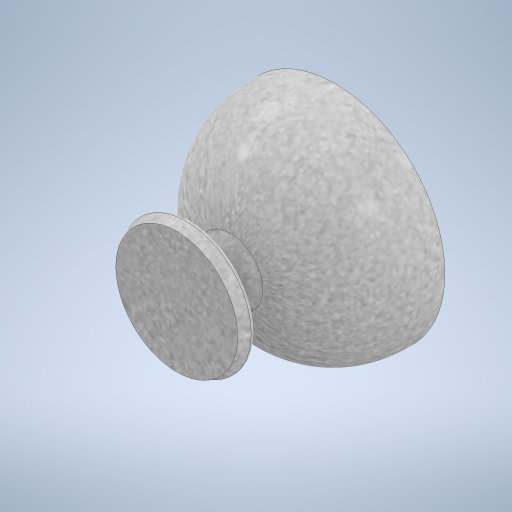
# Autodesk Inventor part: icecup
Saved by Autodesk Inventor 2024 (Build 280153000, 153)
## iProperties
Created: 2024-03-22
Part Number: icecup
Material: Glasfaserbeton
Document SubType Name: Modeling
Designer: ffogue
Density: 1.7 g/cm^3
Appearance: Flach - Poliert Grau
Author: ffogue
Autodesk Inventor part; units mm, degrees
ref_plane "YZ Plane" through (0, 0, 0) normal (1, 0, 0) x (0, 1, 0)
ref_plane "XZ Plane" through (0, 0, 0) normal (0, 1, 0) x (-1, 0, 0)
ref_plane "XY Plane" through (0, 0, 0) normal (0, 0, 1) x (1, 0, 0)
sketch "Skizze1" plane through (0, 0, 0) normal (0, 0, 1) x (1, 0, 0)
  line L0 (0, 0) -> (0, 65)
  line L1 (0, 0) -> (25, 0)
  line L2 (25, 0) -> (26.9847, 5)
  line L3 (26.9847, 5) -> (13.2943, 8.4396)
  arc A0 (13.2943, 22.0176) -> (13.2943, 8.4396) centre (15, 15.2286) ccw
  arc A1 (13.2943, 22.0176) -> (45, 65) centre (3.0602, 62.7517) ccw
  line L4 (45, 65) -> (0, 65)
  line L5 (0, 15.2286) -> (25.9618, 15.2286) construction
  dimension "d0" = 65
  dimension "d3" = 30
  dimension "d4" = 50
  dimension "d5" = 90
  dimension "d6" = 7
  dimension "d7" = 21.65
  dimension "d8" = 42
  dimension "d9" = 5
  constraints: 12 end point, 5 point on circle, 2 centre point, 2 horizontal, 2 tangent, 1 horizontal alignment, 1 perpendicular, 1 point on line, 1 symmetric about line, 1 vertical, 1 vertical alignment
  measures "d0" distance between parallel lines of L1 L4
  measures "d3" diameter of A0.centre L0
  measures "d4" diameter of L1.end L0
  measures "d5" diameter of A1.end L0
  measures "d6" radius of A0
  measures "d7" angle of L2 L0
  measures "d8" radius of A1
  measures "d9" vertical distance of L1.end L2.end
revolve "Umdrehung1" add sketch "Skizze1" angle 360 about axis through (0, 0, 0) along (0, 1, 0)
fillet "Rundung2" radius 1 1 edges at (-26.9847, 5, 0)
shell "Wandung2" thickness 4 removed faces 1 at (12.1353, 65, 8.8168)
